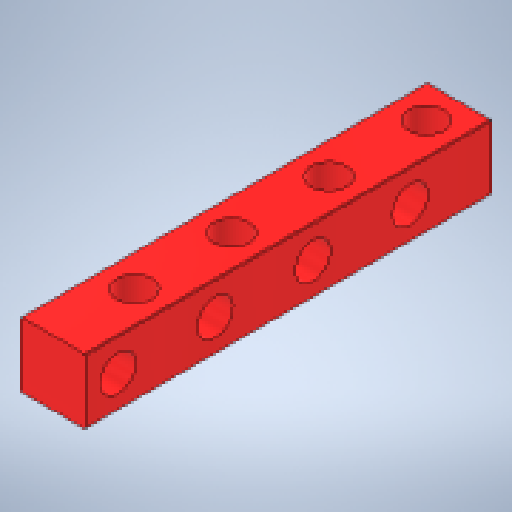
# Autodesk Inventor part: Nut Strip
Saved by Autodesk Inventor 2023.2 (Build 272271000, 271)
## iProperties
Created: 2024-01-21
Part Number: Nut Strip
Material: Aluminum 6061
Document SubType Name: Modeling
Designer: Nathan Cai
Density: 2.7 g/cm^3
Appearance: Light Red
Author: Nathan Cai
Autodesk Inventor part; units mm, degrees
ref_plane "YZ Plane" through (0, 0, 0) normal (1, 0, 0) x (0, 1, 0)
ref_plane "XZ Plane" through (0, 0, 0) normal (0, 1, 0) x (-1, 0, 0)
ref_plane "XY Plane" through (0, 0, 0) normal (0, 0, 1) x (1, 0, 0)
sketch "Sketch1" plane through (0, 0, 0) normal (0, 0, 1) x (1, 0, 0)
  line L0 (-3.175, -3.175) -> (3.175, -3.175)
  line L1 (3.175, -3.175) -> (3.175, 3.175)
  line L2 (3.175, 3.175) -> (-3.175, 3.175)
  line L3 (-3.175, 3.175) -> (-3.175, -3.175)
  line L4 (-3.175, -3.175) -> (3.175, 3.175) construction
  line L5 (3.175, -3.175) -> (-3.175, 3.175) construction
  point P0 (0, 0)
  dimension "d0" = 6.35
  dimension "d1" = 6.35
  constraints: 12 end point, 2 midpoint, 2 parallel, 1 horizontal, 1 perpendicular
  measures "d0" distance of L2.end L1.end
  measures "d1" distance of L1.end L0.end
extrude "Extrusion1" add sketch "Sketch1" along normal blind 39.6875
sketch "Sketch2" plane through (-3.175, 3.175, 0) normal (0, 1, 0) x (1, 0, 0)
  line L0 (3.175, 0) -> (3.175, -39.6875) construction
  line L1 (6.35, -39.6875) -> (0, -39.6875) projected
  circle A0 centre (3.175, -3.175) radius 1.7526
  circle A1 centre (3.175, -12.7) radius 1.7526
  circle A2 centre (3.175, -22.225) radius 1.7526
  circle A3 centre (3.175, -31.75) radius 1.7526
  circle A4 centre (3.175, -36.5125) radius 1.4493 construction
  line L2 (6.35, 0) -> (0, 0) projected
  dimension "d4" = 3.5052
  dimension "d7" = 9.525
  dimension "d12" = 4.7625
  dimension "d13" = 3.175
  constraints: 5 centre point, 2 end point, 2 point on line, 1 midpoint, 1 vertical, 6 other
  measures "d4" diameter of A0
  measures "d7" distance of A0.centre A1.centre
  measures "d12" distance of A3.centre A4.centre
  measures "d13" distance from line of L2 A0.centre
extrude "Extrusion2" cut sketch "Sketch2" against normal through all
sketch "Sketch3" plane through (3.175, -3.175, 0) normal (1, 0, 0) x (0, 0, -1)
  line L0 (0, 3.175) -> (-39.6875, 3.175) construction
  line L1 (-39.6875, 0) -> (-39.6875, 6.35) projected
  circle A0 centre (-36.5125, 3.175) radius 1.7526
  circle A1 centre (-26.9875, 3.175) radius 1.7526
  circle A2 centre (-17.4625, 3.175) radius 1.7526
  circle A3 centre (-7.9375, 3.175) radius 1.7526
  dimension "d16" = 3.5052
  dimension "d17" = 3.175
  dimension "d20" = 9.525
  constraints: 4 centre point, 2 end point, 1 horizontal, 1 midpoint, 1 point on line, 6 other
  measures "d16" diameter of A0
  measures "d17" distance from line of L1 A0.centre
  measures "d20" distance of A0.centre A1.centre
extrude "Extrusion3" cut sketch "Sketch3" against normal through all
chamfer "Chamfer1" distance 0.1 angle 45 4 edges at (-3.175, 3.175, 19.8438) (3.175, 3.175, 19.8438) (3.175, -3.175, 19.8438) (-3.175, -3.175, 19.8438)
body "Solid1"
